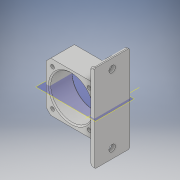
# Autodesk Inventor part: bullog_mount
Saved by Autodesk Inventor 2019 (Build 230136000, 136)
## iProperties
Created: 2018-10-05
Part Number: bullog_mount
Material: Generisch
Document SubType Name: Modeling
Designer: marc
Density: 1 g/cm^3
Appearance: Vorgabe
Author: marc
## iProperties of the stored document bullog_mount_3D-Druck.ipt
Created: 2018-10-05
Part Number: bullog_mount_3D-Druck
Material: Generisch
Document SubType Name: Modeling
Designer: marc
Density: 1 g/cm^3
Appearance: Vorgabe
Author: marc
Autodesk Inventor part; units mm, degrees
ref_plane "YZ Plane" through (0, 0, 0) normal (1, 0, 0) x (0, 1, 0)
ref_plane "XZ Plane" through (0, 0, 0) normal (0, 1, 0) x (-1, 0, 0)
ref_plane "XY Plane" through (0, 0, 0) normal (0, 0, 1) x (1, 0, 0)
sketch "Skizze1" plane through (0, 0, 0) normal (0, 0, 1) x (1, 0, 0)
  line L0 (21, -21) -> (-21, -21)
  line L1 (-21, -21) -> (-21, 21)
  line L2 (-21, 21) -> (21, 21)
  line L3 (21, 21) -> (21, -21)
  line L4 (21, -21) -> (-21, 21) construction
  line L5 (-21, -21) -> (21, 21) construction
  circle A0 centre (0, 0) radius 18
  circle A1 centre (-15.5, 15.5) radius 1.6
  circle A2 centre (15.5, 15.5) radius 1.6
  circle A3 centre (15.5, -15.5) radius 1.6
  circle A4 centre (-15.5, -15.5) radius 1.6
  dimension "d0" = 42
  dimension "d1" = 42
  dimension "d2" = 36
  dimension "d3" = 31
  dimension "d4" = 15.5
  dimension "d5" = 3.2
  dimension "d6" = 3.2
  dimension "d7" = 3.2
  dimension "d8" = 3.2
  constraints: 12 end point, 5 centre point, 5 coincident, 2 midpoint, 2 parallel, 2 point on line, 2 symmetric about line, 1 horizontal, 1 perpendicular, 1 vertical alignment
  measures "d0" distance of L1.end L2.end
  measures "d1" distance of L0.end L1.end
  measures "d2" diameter of A0
  measures "d3" distance of point (15.5, -15.5) point (15.5, 15.5)
  measures "d4" horizontal distance of point (15.5, 15.5) point (0, 0)
  measures "d5" diameter of A1
  measures "d6" diameter of A2
  measures "d7" diameter of A3
  measures "d8" diameter of A4
extrude "Extrusion1" add sketch "Skizze1" along normal blind 20
sketch "Skizze2" plane through (21, -21, 0) normal (1, 0, 0) x (0, 0, -1)
  line L0 (-25, -16) -> (5, -16)
  line L1 (5, -16) -> (5, 58)
  line L2 (5, 58) -> (-25, 58)
  line L3 (-25, 58) -> (-25, -16)
  line L4 (-25, -16) -> (5, 58) construction
  line L5 (5, -16) -> (-25, 58) construction
  line L6 (0, 0) -> (-20, 0) projected
  line L7 (0, 42) -> (-20, 42) projected
  line L8 (0, 42) -> (0, 0) projected
  point P0 (0, 21)
  point P1 (-10, 21)
  point P2 (0, 21)
  dimension "d11" = 30
  dimension "d12" = 74
  dimension "d13" = 42
  dimension "d14" = 20
  dimension "d15" = 10
  dimension "d16" = 21
  constraints: 12 end point, 3 midpoint, 2 parallel, 1 horizontal, 1 horizontal alignment, 1 perpendicular
  measures "d11" distance of L2.end L1.end
  measures "d12" distance of L0.end L1.end
  measures "d13" distance between parallel lines of L6 L7
  measures "d14" distance of L7.start L7.end
  measures "d15" distance of point (0, 21) point (-10, 21)
  measures "d16" distance from line of point (-10, 21) L7
extrude "Extrusion2" add sketch "Skizze2" along normal blind 4
sketch "Skizze3" plane through (21, -21, 0) normal (-1, 0, 0) x (0, 0, 1)
  line L0 (0, 0) -> (20, 0) projected
  line L1 (25, -16) -> (-5, -16) projected
  line L2 (25, 58) -> (25, -16) projected
  point P0 (0, 21)
  point P1 (10, -8)
  dimension "d19" = 16
  dimension "d20" = 15
  dimension "d21" = 30
  dimension "d22" = 8
  measures "d19" distance between parallel lines of L0 L1
  measures "d20" distance from line of L2 point (10, -8)
  measures "d21" distance of L1.start L1.end
  measures "d22" distance from line of L1 point (10, -8)
hole "Bohrung1" at (21, -29, 10) direction (1, 0, 0) diameter 5.5 end through all counterbore diameter 15 counterbore depth 1 clearance for "Sechskantkopfschraube DIN EN 24017" size "M5" standard "DIN"
ref_plane "Arbeitsebene1" through (21, 0, -5) normal (0, -1, 0) x (0, 0, -1)
mirror "Spiegeln1" about plane through (21, 0, -5) normal (0, -1, 0) of "Bohrung1"
chamfer "Fase1" distance 4 angle 45 2 edges at (-21, -21, 10) (-21, 21, 10)
fillet "Rundung1" radius 2 4 edges at (21, 0, 20) (21, -21, 10) (21, 21, 10) (21, 0, 0)
fillet "Rundung2" radius 3 2 edges at (21, -37, 10) (21, 37, 10)
chamfer "Fase2" distance 1 angle 45 10 edges at (21, 0, 25) (21.8787, -36.1213, 25) (24.5, -37, 25) (21.8787, 36.1213, 25) (24.5, 37, 25) (21, 0, -5) (21.8787, 36.1213, -5) (24.5, 37, -5) (21.8787, -36.1213, -5) (24.5, -37, -5)
chamfer "Fase3" distance 1 angle 45 2 edges at (-18, 0, 20) (-18, 0, 0)
equation "\"d1\" = d0"
equation "\"d6\" = d5"
equation "\"d15\" = 0.5 * d14"
equation "\"d20\" = 0.5 * d21"
equation "\"d22\" = 0.5 * d19"
